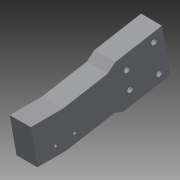
# Autodesk Inventor part: Arm_Link_1
Saved by Autodesk Inventor 2013 (Build 170138000, 138)
## iProperties
Created: 2014-05-15
Part Number: Arm_Link_1
Material: 一般
Document SubType Name: Modeling
Designer: andou
Density: 1 g/cm^3
Author: andou
Autodesk Inventor part; units mm, degrees
ref_plane "YZ Plane" through (0, 0, 0) normal (1, 0, 0) x (0, 1, 0)
ref_plane "XZ Plane" through (0, 0, 0) normal (0, 1, 0) x (-1, 0, 0)
ref_plane "XY Plane" through (0, 0, 0) normal (0, 0, 1) x (1, 0, 0)
sketch "スケッチ2" plane through (0, 0, 0) normal (1, 0, 0) x (0, 1, 0)
  line L0 (0, 0) -> (-49.3161, 0)
  line L1 (-49.3161, -20) -> (1.7498, -20)
  line L2 (0, 0) -> (48.5669, 8.5637)
  line L3 (52.0398, -11.1325) -> (1.7498, -20)
  arc A0 (52.6511, 8.4361) -> (48.5669, 8.5637) centre (50.3034, -1.2844) ccw
  arc A1 (52.0398, -11.1325) -> (55.8341, -9.6157) centre (50.3034, -1.2844) ccw
  arc A2 (-53.3161, -19.1652) -> (-49.3161, -20) centre (-49.3161, -10) ccw
  arc A3 (-49.3161, 0) -> (-53.3161, -0.8348) centre (-49.3161, -10) ccw
  arc A4 (-49.3161, -14) -> (-49.3161, -6) centre (-49.3161, -10) ccw
  line L4 (-49.3161, -6) -> (-53.3161, -6)
  line L5 (-49.3161, -14) -> (-53.3161, -14)
  line L6 (-53.3161, -0.8348) -> (-53.3161, -6)
  line L7 (-53.3161, -14) -> (-53.3161, -19.1652)
  line L8 (52.6511, 8.4361) -> (53.548, 3.3494)
  line L9 (54.9372, -4.5291) -> (55.8341, -9.6157)
  line L10 (1.7498, -20) -> (0, 0)
  line L11 (53.548, 3.3494) -> (54.9372, -4.5291)
  dimension "d21" = 20
  dimension "d22" = 10
  dimension "d23" = 170
  dimension "d25" = 10
  dimension "d27" = 10
  dimension "d31" = 8
  dimension "d33" = 4
  dimension "d35" = 4
  dimension "d36" = 100
  constraints: 24 end point, 10 point on circle, 8 perpendicular, 5 centre point, 4 equal length, 3 equal radius, 2 parallel, 2 tangent, 1 coincident, 1 collinear, 1 horizontal
  measures "d21" distance between parallel lines of L0 L1
  measures "d22" distance from line of L0 A2.centre
  measures "d23" angle of L0 L2
  measures "d25" distance from line of L3 A0.centre
  measures "d27" radius of A3
  measures "d31" diameter of A4
  measures "d33" distance from line of L6 A2.centre
  measures "d35" distance from line of L8 L2.end
  measures "d36" distance of A2.centre A0.centre
extrude "押し出し1" add sketch "スケッチ2" along normal blind 11
sketch "スケッチ4" plane through (0, 0, 0) normal (-1, 0, 0) x (0, 0, 1)
  line L0 (-20, 1.7498) -> (-11.1325, 52.0398) projected
  line L1 (-20, -49.3161) -> (-20, 1.7498) projected
  circle A0 centre (-15, -3.7068) radius 1
  circle A1 centre (-14.1284, 6.2552) radius 1
  line L2 (-15, -3.7068) -> (-14.1284, 6.2552)
  dimension "d57" = 2
  dimension "d59" = 10
  dimension "d60" = 175
  dimension "d61" = 5
  dimension "d62" = 5
  constraints: 2 centre point, 2 end point, 1 equal radius
  measures "d57" diameter of A0
  measures "d59" distance of L2.start L2.end
  measures "d60" angle of L1 L2
  measures "d61" distance from line of L1 L2.start
  measures "d62" distance from line of L0 L2.end
hole "穴2" at (0, -3.7068, -15) at (0, 6.2552, -14.1284) direction (1, 0, 0) diameter 1.6 end through all
sketch "スケッチ6" plane through (11, 0, 0) normal (1, 0, 0) x (0, 0, -1)
  line L0 (20, 1.7498) -> (11.1325, 52.0398) projected
  arc A0 (11.1325, 52.0398) -> (9.6157, 55.8341) centre (1.2844, 50.3034) ccw projected
  line L1 (9.6157, 55.8341) -> (-8.4361, 52.6511) projected
  arc A1 (-8.4361, 52.6511) -> (-8.5637, 48.5669) centre (1.2844, 50.3034) ccw projected
  line L2 (-8.5637, 48.5669) -> (0, 0) projected
  line L3 (-4.1651, 23.6216) -> (-7.3791, 27.4518)
  line L4 (-8.4361, 52.6511) -> (-11.7203, 52.072)
  line L5 (-11.7203, 52.072) -> (-7.3791, 27.4518)
  line L6 (9.6157, 55.8341) -> (12.8999, 56.4132)
  line L7 (12.8999, 56.4132) -> (17.2411, 31.793)
  line L8 (17.2411, 31.793) -> (15.531, 27.0945)
  dimension "d75" = 150
  dimension "d76" = 150
  dimension "d77" = 2.5
  dimension "d78" = 2.5
  dimension "d79" = 25
  constraints: 12 end point, 3 parallel, 2 collinear, 2 point on line
  measures "d75" angle of L2 L3
  measures "d76" angle of L0 L8
  measures "d77" distance between parallel lines of L0 L7
  measures "d78" distance between parallel lines of L2 L5
  measures "d79" distance of L4.end L3.end
extrude "押し出し2" add sketch "スケッチ6" against normal blind 11
sketch "スケッチ5" plane through (11, 0, 0) normal (1, 0, 0) x (0, 0, -1)
  line L0 (9.6157, 55.8341) -> (-8.4361, 52.6511) projected
  line L1 (-8.5637, 48.5669) -> (0, 0) projected
  circle A0 centre (-6.4204, 47.9294) radius 1.5
  circle A1 centre (9.3365, 50.7077) radius 1.5
  line L2 (15.531, 27.0945) -> (20, 1.7498) projected
  line L3 (20, 1.7498) -> (20, -49.3161) projected
  arc A2 (19.1652, -53.3161) -> (20, -49.3161) centre (10, -49.3161) ccw projected
  line L4 (19.1652, -53.3161) -> (14, -53.3161) projected
  line L5 (14, -53.3161) -> (14, -49.3161) projected
  arc A3 (14, -49.3161) -> (6, -49.3161) centre (10, -49.3161) ccw projected
  line L6 (6, -49.3161) -> (6, -53.3161) projected
  line L7 (6, -53.3161) -> (0.8348, -53.3161) projected
  arc A4 (0, -49.3161) -> (0.8348, -53.3161) centre (10, -49.3161) ccw projected
  line L8 (0, -49.3161) -> (0, 0) projected
  line L9 (0, 0) -> (-4.1651, 23.6216) projected
  circle A5 centre (15, -3.7068) radius 0.8 projected
  circle A6 centre (14.1284, 6.2552) radius 0.8 projected
  line L10 (-7.3791, 27.4518) -> (-11.7203, 52.072) projected
  line L11 (-11.7203, 52.072) -> (12.8999, 56.4132) projected
  line L12 (12.8999, 56.4132) -> (17.2411, 31.793) projected
  line L13 (17.2411, 31.793) -> (15.531, 27.0945) projected
  line L14 (-4.1651, 23.6216) -> (-7.3791, 27.4518) projected
  dimension "d70" = 5
  dimension "d71" = 5
  dimension "d72" = 3
  dimension "d73" = 16
  dimension "d74" = 2
  constraints: 2 centre point, 1 equal radius
  measures "d70" distance from line of L0 A0.centre
  measures "d71" distance from line of L0 A1.centre
  measures "d72" diameter of A1
  measures "d73" distance of A1.centre A0.centre
  measures "d74" distance from line of L1 A0.centre
hole "穴3" at (11, 47.9294, 6.4204) at (11, 50.7077, -9.3365) direction (-1, 0, 0) diameter 3 end through all
sketch "スケッチ7" plane through (11, 0, 0) normal (1, 0, 0) x (0, 0, -1)
  arc A0 (0, -49.3161) -> (0.8348, -53.3161) centre (10, -49.3161) ccw projected
  line L0 (0.8348, -53.3161) -> (6, -53.3161) projected
  circle A1 centre (3, -49.3161) radius 1
  dimension "d89" = 4
  dimension "d90" = 7
  dimension "d91" = 2
  constraints: 1 centre point
  measures "d89" distance from line of L0 A1.centre
  measures "d90" distance of A1.centre A0.centre
  measures "d91" diameter of A1
hole "穴4" at (11, -49.3161, -3) direction (-1, 0, 0) diameter 2 end through all
pattern_circular "円形状パターン3" count 5 over 180 about axis through (0, -49.3161, -10) along (-1, 0, 0) of "穴4"
sketch "スケッチ8" plane through (11, 0, 0) normal (1, 0, 0) x (0, 0, -1)
  line L0 (12.8999, 56.4132) -> (-11.7203, 52.072) projected
  line L1 (-11.7203, 52.072) -> (-7.3791, 27.4518) projected
  circle A0 centre (-0.8612, 33.6782) radius 1.5
  circle A1 centre (8.9868, 35.4147) radius 1.5
  dimension "d102" = 3
  dimension "d104" = 20
  dimension "d105" = 20
  dimension "d106" = 10
  dimension "d107" = 7.5
  constraints: 2 centre point, 1 equal radius
  measures "d102" diameter of A0
  measures "d104" distance from line of L0 A0.centre
  measures "d105" distance from line of L0 A1.centre
  measures "d106" distance of A1.centre A0.centre
  measures "d107" distance from line of L1 A0.centre
hole "穴5" at (11, 33.6782, 0.8612) at (11, 35.4147, -8.9868) direction (-1, 0, 0) diameter 3 end through all
sketch "スケッチ9" plane through (11, 0, 0) normal (1, 0, 0) x (0, 0, -1)
  circle A0 centre (-0.8612, 33.6782) radius 1.5 projected
  circle A1 centre (8.9868, 35.4147) radius 1.5 projected
  circle A2 centre (-6.4204, 47.9294) radius 1.5 projected
  circle A3 centre (9.3365, 50.7077) radius 1.5 projected
  circle A4 centre (15, -3.7068) radius 0.8 projected
  circle A5 centre (14.1284, 6.2552) radius 0.8 projected
  line L0 (0, 0) -> (0, -49.3161) projected
  line L1 (20, -49.3161) -> (20, 1.7498) projected
  line L2 (20, 1.7498) -> (15.531, 27.0945) projected
  line L3 (15.531, 27.0945) -> (17.2411, 31.793) projected
  line L4 (17.2411, 31.793) -> (12.8999, 56.4132) projected
  line L5 (12.8999, 56.4132) -> (-11.7203, 52.072) projected
  line L6 (-11.7203, 52.072) -> (-7.3791, 27.4518) projected
  line L7 (-7.3791, 27.4518) -> (-4.1651, 23.6216) projected
  line L8 (-4.1651, 23.6216) -> (0, 0) projected
  line L9 (0, -16.9413) -> (20, -13.4147)
  dimension "d115" = 70
  constraints: 2 end point, 2 point on line, 1 parallel
  measures "d115" distance between parallel lines of L5 L9
extrude "押し出し3" cut sketch "スケッチ9" against normal blind 11 keep common part
